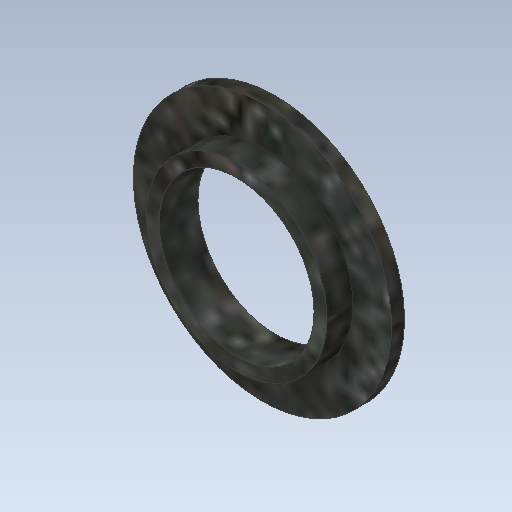
# Autodesk Inventor part: ドライメット　内径12 フランジ付き2mm
Saved by Autodesk Inventor 2020.2 (Build 242310000, 310)
## iProperties
Created: 2019-11-09
Part Number: ドライメット　内径12 フランジ付き2mm
Material: 鋼
Document SubType Name: Modeling
Designer: mozar
Density: 7.85 g/cm^3
Appearance: プレート
Mass: 2.21954 g
Surface Area: 6.66018 cm^2
Volume: 0.282743 cm^3
Author: mozar
Autodesk Inventor part; units mm, degrees
ref_plane "YZ Plane" through (0, 0, 0) normal (1, 0, 0) x (0, 1, 0)
ref_plane "XZ Plane" through (0, 0, 0) normal (0, 1, 0) x (-1, 0, 0)
ref_plane "XY Plane" through (0, 0, 0) normal (0, 0, 1) x (1, 0, 0)
sketch "スケッチ1" plane through (0, 0, 0) normal (0, 0, 1) x (1, 0, 0)
  circle A0 centre (0, 0) radius 6
  circle A1 centre (0, 0) radius 7
  circle A2 centre (0, 0) radius 10
  dimension "d0" = 12
  dimension "d1" = 14
  dimension "d2" = 20
  constraints: 3 centre point, 3 coincident
  measures "d0" diameter of A0
  measures "d1" diameter of A1
  measures "d2" diameter of A2
extrude "押し出し1" add sketch "スケッチ1" along normal blind 2 contours A1
extrude "押し出し2" add sketch "スケッチ1" against normal blind 1 contours A1 | A2
